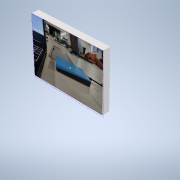
# Autodesk Inventor part: SXS
Saved by Autodesk Inventor 2022 (Build 260153000, 153)
## iProperties
Created: 2022-02-04
Part Number: SXS
Material: Generic
Document SubType Name: Modeling
Designer: joshw
Density: 1 g/cm^3
Appearance: Default
Author: joshw
Autodesk Inventor part; units mm, degrees
ref_plane "YZ Plane" through (0, 0, 0) normal (1, 0, 0) x (0, 1, 0)
ref_plane "XZ Plane" through (0, 0, 0) normal (0, 1, 0) x (-1, 0, 0)
ref_plane "XY Plane" through (0, 0, 0) normal (0, 0, 1) x (1, 0, 0)
sketch "Sketch1" plane through (0, 0, 0) normal (0, 0, 1) x (1, 0, 0)
  line L0 (-148.007302, 104.602631) -> (122.92604, 104.602631) construction
  line L1 (122.92604, 104.602631) -> (122.92604, -98.597366) construction
  line L2 (122.92604, -98.597366) -> (-148.007302, -98.597366) construction
  line L3 (-148.007302, -98.597366) -> (-148.007302, 104.602631) construction
  point P0 (0, 0)
  constraints: 2 other
sketch "Sketch3" plane through (0, 0, 0) normal (0, 0, 1) x (1, 0, 0)
  line L0 (-147.399591, 106.795076) -> (122.868294, 106.795076) construction
  line L1 (122.868294, 106.795076) -> (122.868294, -95.905826) construction
  line L2 (122.868294, -95.905826) -> (-147.399591, -95.905826) construction
  line L3 (-147.399591, -95.905826) -> (-147.399591, 106.795076) construction
  point P0 (0, 0)
  constraints: 2 other
sketch "Sketch4" plane through (0, 0, 0) normal (0, 0, 1) x (1, 0, 0)
  line L0 (-147.34869, 106.970933) -> (120.2293, 106.970933)
  line L1 (120.2293, 106.970933) -> (120.2293, -94.315217)
  line L2 (120.2293, -94.315217) -> (-147.34869, -94.315217)
  line L3 (-147.34869, -94.315217) -> (-147.34869, 106.970933)
  point P0 (0, 0)
  constraints: 8 end point, 2 parallel, 1 horizontal, 1 perpendicular
extrude "Extrusion2" add sketch "Sketch4" against normal blind 25.4
sketch "Sketch5" plane through (0, 0, 0) normal (0, 0, 1) x (1, 0, 0)
  line L0 (-147.34869, -94.315217) -> (120.2293, -94.315217)
  line L1 (120.2293, -94.315217) -> (120.2293, 106.970933)
  line L2 (120.2293, 106.970933) -> (-147.34869, 106.970933)
  line L3 (-147.34869, 106.970933) -> (-147.34869, -94.315217)
  point P0 (0, 0)
extrude "Extrusion3" cut sketch "Sketch5" against normal blind 0.000025
decal "Decal1"
body "Solid2"
